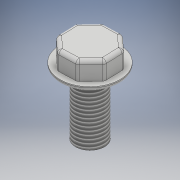
# Autodesk Inventor part: AnnishNT
Saved by Autodesk Inventor 2017 (Build 210142000, 142)
## iProperties
Created: 2018-02-22
Part Number: AnnishNT
Material: Generic
Document SubType Name: Modeling
Designer: CMRU-CAD-PC 7
Density: 1 g/cm^3
Appearance: Default
Author: CMRU-CAD-PC 7
Autodesk Inventor part; units mm, degrees
ref_plane "YZ Plane" through (0, 0, 0) normal (1, 0, 0) x (0, 1, 0)
ref_plane "XZ Plane" through (0, 0, 0) normal (0, 1, 0) x (-1, 0, 0)
ref_plane "XY Plane" through (0, 0, 0) normal (0, 0, 1) x (1, 0, 0)
sketch "Sketch1" plane through (0, 0, 0) normal (0, 0, 1) x (1, 0, 0)
  line L0 (13.1171, -4.9434) -> (5.7797, -12.7707)
  line L1 (5.7797, -12.7707) -> (-4.9434, -13.1171)
  line L2 (-4.9434, -13.1171) -> (-12.7707, -5.7797)
  line L3 (-12.7707, -5.7797) -> (-13.1171, 4.9434)
  line L4 (-13.1171, 4.9434) -> (-5.7797, 12.7707)
  line L5 (-5.7797, 12.7707) -> (4.9434, 13.1171)
  line L6 (4.9434, 13.1171) -> (12.7707, 5.7797)
  line L7 (12.7707, 5.7797) -> (13.1171, -4.9434)
  point P0 (0, 0)
  point P1 (0, 0)
  constraints: 16 end point, 1 coincident, 17 other
extrude "Extrusion1" add sketch "Sketch1" along normal blind 10
fillet "Fillet1" radius 2 15 edges at (-0.4182, 12.9439, 10) (4.9434, 13.1171, 5) (-5.7797, 12.7707, 5) (12.7707, 5.7797, 5) (8.857, 9.4484, 10) (13.1171, -4.9434, 5) (12.9439, 0.4182, 10) (5.7797, -12.7707, 5) (9.4484, -8.857, 10) (-4.9434, -13.1171, 5) (0.4182, -12.9439, 10) (-12.7707, -5.7797, 5) (-8.857, -9.4484, 10) (-12.9439, -0.4182, 10) (-9.4484, 8.857, 10)
sketch "Sketch2" plane through (0, 0, 0) normal (0, 0, -1) x (-1, 0, 0)
  circle A0 centre (0, 0) radius 16.569
  constraints: 1 centre point, 1 coincident
extrude "Extrusion2" add sketch "Sketch2" along normal blind 2.6
fillet "Fillet2" radius 2 1 edges at (16.569, 0, -2.6)
sketch "Sketch3" plane through (0, 0, -2.6) normal (0, 0, -1) x (-1, 0, 0)
  circle A0 centre (0, 0) radius 8
  dimension "d7" = 16
  constraints: 1 centre point, 1 coincident
  measures "d7" diameter of A0
extrude "Extrusion3" add sketch "Sketch3" along normal blind 34
thread "Thread1" size "M16x2" class "6g" standard "ISO Metric profile" full length
body "Solid1"
